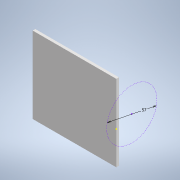
# Autodesk Inventor part: Palma
Saved by Autodesk Inventor 2020.4 (Build 244396010, 396A)
## iProperties
Created: 2021-09-01
Part Number: Palma
Material: Generic
Document SubType Name: Modeling
Designer: chalo
Density: 1 g/cm^3
Appearance: Default
Author: chalo
Autodesk Inventor part; units mm, degrees
ref_plane "YZ Plane" through (0, 0, 0) normal (1, 0, 0) x (0, 1, 0)
ref_plane "XZ Plane" through (0, 0, 0) normal (0, 1, 0) x (-1, 0, 0)
ref_plane "XY Plane" through (0, 0, 0) normal (0, 0, 1) x (1, 0, 0)
sketch "Sketch1" plane through (0, 0, 0) normal (0, 0, 1) x (1, 0, 0)
  line L0 (-4.4, 49.4) -> (30, 49.4) projected
  line L1 (-4.4, -37.6) -> (30, -37.6) projected
  line L2 (-4.4, -37.6) -> (90.6, -37.6)
  line L3 (90.6, -37.6) -> (90.6, 49.4)
  line L4 (90.6, 49.4) -> (-4.4, 49.4)
  line L5 (-4.4, 49.4) -> (-4.4, -37.6)
  point P0 (0, 0)
  dimension "d0" = 95
  constraints: 8 end point, 2 parallel, 1 horizontal, 1 perpendicular
  measures "d0" distance of L0.start L3.end
extrude "Extrusion1" add sketch "Sketch1" against normal blind 3
sketch "Sketch2" plane through (90.6, -37.6, 0) normal (1, 0, 0) x (0, 0, -1)
  circle A0 centre (17.5922, 43.5) radius 28.5 construction
  point P0 (0, 37.6)
  dimension "d5" = 57
  constraints: 1 centre point
  measures "d5" diameter of A0
sketch "Sketch3" plane through (0, 0, 0) normal (0, 0, 1) x (1, 0, 0)
  line L0 (90.6, 49.4) -> (-4.4, 49.4) projected
  line L1 (-4.4, 49.4) -> (-4.4, -37.6) projected
  line L2 (-4.4, -37.6) -> (90.6, -37.6) projected
  line L3 (90.6, -37.6) -> (90.6, 49.4) projected
  line L4 (90.6, 49.4) -> (-4.4, 49.4) projected
  line L5 (-4.4, 49.4) -> (90.6, 49.4) projected
  arc A0 (25.8108, 49.4) -> (78.1488, 49.4) centre (51.9798, 64.0691) ccw
  point P0 (0, 0)
  point P1 (25.8108, 49.4)
  point P2 (78.1488, 49.4)
  dimension "d9" = 30
  constraints: 2 point on circle, 2 point on line, 1 centre point
  measures "d9" radius of A0
extrude "Extrusion2" add sketch "Sketch3" along normal blind 15 contours A0 L0
sketch "Sketch4" plane through (-4.4, 49.4, -3) normal (0, 1, 0) x (1, 0, 0)
  point P0 (4.4, -3)
fillet "Fillet2" radius 10 2 edges at (51.9798, 34.0691, 15) (51.9798, 34.0691, 0)
sketch "Sketch7" plane through (0, 0, -3) normal (0, 0, -1) x (-1, 0, 0)
  line L0 (4.4, 49.4) -> (-90.6, 49.4) projected
  line L1 (-90.6, 49.4) -> (-90.6, -37.6) projected
  line L2 (-90.6, -37.6) -> (4.4, -37.6) projected
  line L3 (4.4, -37.6) -> (4.4, 49.4) projected
  line L4 (-90.6, -37.6) -> (4.4, -37.6) projected
  arc A0 (-90.6, -30.1) -> (-60.6, -37.6) centre (-60.6, 26.15) ccw
  line L5 (-90.6, 49.4) -> (-90.6, -37.6) projected
  line L6 (-90.6, 5.9) -> (-40.6, 5.9) construction
  arc A1 (-60.6, 49.4) -> (-90.6, 41.9) centre (-60.6, -14.35) ccw
  point P0 (0, 0)
  point P1 (-60.6, -37.6)
  dimension "d11" = 30
  dimension "d12" = 7.5
  dimension "d13" = 50
  constraints: 4 point on circle, 3 symmetric about line, 2 centre point, 2 end point, 2 point on line, 1 horizontal, 1 midpoint, 1 tangent, 1 other
  measures "d11" distance of L1.end A0.end
  measures "d12" distance of L1.end A0.start
  measures "d13" distance of L6.start L6.end
extrude "Extrusion3" cut sketch "Sketch7" against normal through all contours A1 L1 L0 | L2 L1 A0
sketch "Sketch8" plane through (0, 0, -3) normal (0, 0, -1) x (-1, 0, 0)
  arc A0 (-60.6, 49.4) -> (-90.6, 41.9) centre (-60.6, -14.35) ccw projected
  line L0 (-90.6, 41.9) -> (-90.6, -30.1) projected
  arc A1 (-90.6, -30.1) -> (-60.6, -37.6) centre (-60.6, 26.15) ccw projected
  line L1 (-60.6, -37.6) -> (4.4, -37.6) projected
  line L2 (4.4, -37.6) -> (4.4, 49.4) projected
  line L3 (4.4, 49.4) -> (-60.6, 49.4) projected
  arc A2 (-90.6, -30.1) -> (-60.6, -37.6) centre (-60.6, 26.15) ccw projected
  arc A3 (-90.6, 41.9) -> (-90.6, -30.1) centre (-71.4, 5.9) ccw
  point P0 (0, 0)
  constraints: 2 point on circle, 1 centre point, 1 tangent
extrude "Extrusion4" add sketch "Sketch8" against normal blind 3 contours L0 A3
sketch "Sketch9" plane through (0, 0, -3) normal (0, 0, -1) x (-1, 0, 0)
  line L0 (-52.7475, -27.5099) -> (-72.7475, -27.5099)
  line L1 (-72.7475, -27.5099) -> (-72.7475, -34.5099)
  line L2 (-72.7475, -34.5099) -> (-52.7475, -34.5099)
  line L3 (-52.7475, -34.5099) -> (-52.7475, -27.5099)
  line L4 (4.4, -37.6) -> (4.4, 49.4) projected
  line L5 (4.4, 5.9) -> (-145.6, 5.9) construction
  line L6 (-52.7475, 39.3099) -> (-72.7475, 39.3099)
  line L7 (-72.7475, 39.3099) -> (-72.7475, 46.3099)
  line L8 (-72.7475, 46.3099) -> (-52.7475, 46.3099)
  line L9 (-52.7475, 46.3099) -> (-52.7475, 39.3099)
  point P0 (0, 0)
  dimension "d19" = 20
  dimension "d20" = 7
  dimension "d21" = 150
  constraints: 18 end point, 4 symmetric about line, 2 horizontal, 2 parallel, 1 midpoint, 1 perpendicular
  measures "d19" distance of L1.end L2.end
  measures "d20" distance of L0.end L1.end
  measures "d21" distance of L5.start L5.end
extrude "Extrusion5" add sketch "Sketch9" along normal blind 20
sketch "Sketch10" plane through (0, 0, 0) normal (0, 0, 1) x (1, 0, 0)
  line L0 (0.15, 35.15) -> (22.95, 35.15) projected
  line L1 (6.4671, 26.3395) -> (10.4671, 29.307) projected
  line L2 (-4.4, 32.9) -> (30, 32.9) projected
  arc A0 (90.6, 41.9) -> (85.9332, 44.1503) centre (60.6, -14.35) ccw projected
  line L3 (15.4501, 49.4) -> (-4.4, 49.4) projected
  line L4 (-4.4, 49.4) -> (-4.4, -37.6) projected
  line L5 (-4.4, -37.6) -> (60.6, -37.6) projected
  arc A1 (60.6, -37.6) -> (90.6, -30.1) centre (60.6, 26.15) ccw projected
  arc A2 (90.6, -30.1) -> (90.6, 41.9) centre (71.4, 5.9) ccw projected
  line L6 (-4.4, 49.4) -> (60.6, 49.4) projected
  arc A3 (3.8712, 49.4) -> (-4.4, 18.2775) centre (37.3788, 23.8346) ccw
  line L7 (60.6, -37.6) -> (-4.4, -37.6) projected
  arc A4 (-4.4, 18.2775) -> (19.2096, -37.6) centre (64.8355, 14.6046) ccw
  point P0 (0, 0)
  constraints: 4 point on circle, 3 point on line, 2 centre point, 1 other
body "Solid1"
